Autodesk Fusion 360 part; units mm, degrees
note: some values were not read from the file. Set by a fixed rule: which face or edge a step refers to.
(part 3 of 3)
sketch "Sketch2 (4)" plane through (0, 0, 136) normal (0, 0, 1) x (-1, 0, 0) in component "FrontGlass"
  line L0 (-260.8, 5.2) -> (-260.8, 3)
  line L1 (-260.8, 3) -> (-1.2, 3)
  line L2 (-1.2, 3) -> (-1.2, 5.2)
  line L3 (-1.2, 5.2) -> (-260.8, 5.2)
  line L4 (-260.8, 5.2) -> (-250.8, 5.2) construction
  line L5 (-250.8, 5.2) -> (-248.8, 5.2)
  line L6 (-248.8, 5.2) -> (-248.8, 3)
  line L7 (-248.8, 3) -> (-250.8, 3)
  line L8 (-250.8, 3) -> (-250.8, 5.2)
  line L9 (-1.2, 5.2) -> (-11.2, 5.2) construction
  line L10 (-171.6, 3) -> (-171.6, 5.2)
  line L11 (-171.6, 5.2) -> (-169.6, 5.2)
  line L12 (-169.6, 5.2) -> (-169.6, 3)
  line L13 (-169.6, 3) -> (-171.6, 3)
  line L14 (-92.4, 3) -> (-92.4, 5.2)
  line L15 (-92.4, 5.2) -> (-90.4, 5.2)
  line L16 (-90.4, 5.2) -> (-90.4, 3)
  line L17 (-90.4, 3) -> (-92.4, 3)
  line L18 (-13.2, 3) -> (-13.2, 5.2)
  line L19 (-13.2, 5.2) -> (-11.2, 5.2)
  line L20 (-11.2, 5.2) -> (-11.2, 3)
  line L21 (-11.2, 3) -> (-13.2, 3)
  dimension "d328" = 10
  dimension "d329" = 2
  dimension "d330" = 10
  dimension "d348" = 237.6
  dimension "d349" = 0
  constraint perpendicular L0 L4
  constraint horizontal L5
  constraint vertical L6
  constraint horizontal L7
  constraint vertical L8
  constraint collinear L1 L7
  constraint parallel L3 L9
  constraint coincident L2.end L3.start
  constraint coincident L0.start L3.end
  measures "d328" distance of L0.start L4.end
  measures "d329" distance of L4.end L5.end
  measures "d330" distance of L2.end L9.end
extrude "Extrude2''" add sketch "Sketch2 (4)" along normal blind 1.5 contours L1 L3 L5 L6 L7 L8 | L1 L3 L10 L11 L12 L13 | L1 L3 L14 L15 L16 L17 | L1 L3 L18 L19 L20 L21 bodies 18 in component "FrontGlass"
ref_plane "WorkPlane1" through (131, -4.1, 67.5) normal (0, 0, 1) x (1, 0, 0) in component "FrontGlass"
ref_plane "WorkPlane2" through (131, -4.1, 67.5) normal (1, 0, 0) x (0, 0, -1) in component "FrontGlass"
mirror "Mirror1'" about plane through (131, -4.1, 67.5) normal (0, 0, 1) of "Extrude2''" in component "FrontGlass"
sketch "Sketch3 (4)" plane through (-1, 0, 0) normal (-1, 0, 0) x (0, -1, 0) in component "FrontGlass"
  line L0 (3, 1.2) -> (5.2, 1.2)
  line L1 (5.2, 1.2) -> (5.2, 133.8)
  line L2 (5.2, 133.8) -> (3, 133.8)
  line L3 (3, 133.8) -> (3, 1.2)
  line L4 (5.2, 133.8) -> (5.2, 123.8) construction
  line L5 (5.2, 123.8) -> (3, 123.8)
  line L6 (3, 123.8) -> (3, 121.8)
  line L7 (3, 121.8) -> (5.2, 121.8)
  line L8 (5.2, 121.8) -> (5.2, 123.8)
  line L9 (5.2, 1.2) -> (5.2, 11.2) construction
  line L10 (5.2, 11.2) -> (3, 11.2)
  line L11 (3, 11.2) -> (3, 13.2)
  line L12 (3, 13.2) -> (5.2, 13.2)
  line L13 (5.2, 13.2) -> (5.2, 11.2)
  line L14 (5.2, 121.8) -> (5.2, 13.2) construction
  line L15 (5.2, 68.5) -> (3, 68.5)
  line L16 (3, 68.5) -> (3, 66.5)
  line L17 (3, 66.5) -> (5.2, 66.5)
  line L18 (5.2, 66.5) -> (5.2, 68.5)
  dimension "d335" = 10
  dimension "d336" = 2
  dimension "d337" = 10
  dimension "d338" = 2
  dimension "d341" = 2
  constraint perpendicular L2 L4
  constraint horizontal L5
  constraint vertical L6
  constraint horizontal L7
  constraint vertical L8
  constraint coincident L3 L6.end
  constraint perpendicular L0 L9
  constraint horizontal L10
  constraint vertical L11
  constraint horizontal L12
  constraint vertical L13
  constraint coincident L3 L11.end
  constraint horizontal L15
  constraint vertical L16
  constraint horizontal L17
  constraint vertical L18
  constraint coincident L3 L16.end
  constraint coincident L14 L15.start
  constraint midpoint L3 L16
  constraint coincident L0.end L1.start
  constraint coincident L1.end L2.start
  measures "d335" distance of L1.end L4.end
  measures "d336" distance of L4.end L7.end
  measures "d337" distance of L0.end L9.end
  measures "d338" distance of L9.end L12.end
  measures "d341" distance of L15.start L17.end
extrude "Extrude3'''" add sketch "Sketch3 (4)" along normal blind 1.5 contours L1 L3 L10 L11 L12 L13 | L1 L3 L15 L16 L17 L18 | L1 L3 L5 L6 L7 L8 bodies 18 in component "FrontGlass"
mirror "Mirror2''" about plane through (131, -4.1, 67.5) normal (1, 0, 0) of "Extrude3'''" in component "FrontGlass"
combine "Combine9" operation cut target body 15 tool bodies 18 keep tools in component "Enclosure"
combine "Combine10" operation cut target body 14 tool bodies 18 keep tools in component "Enclosure"
combine "Combine11" operation cut target body 16 tool bodies 18 keep tools in component "Enclosure"
combine "Combine12" operation cut target body 13 tool bodies 18 keep tools in component "Enclosure"
move_face "OffsetFaces6" offset -0.1 56 faces at (249.4667, -3, 137) (249.4667, -4.4667, 137.5) (248.8, -4.4667, 136.5) (250.8, -3.7333, 136.5) (170.2667, -3, 136.5) (171.6, -3.7333, 136.5) (170.2667, -4.4667, 137.5) (169.6, -4.4667, 136.5) (90.4, -4.4667, 136.5) (91.0667, -3, 136.5) (91.7333, -3.7333, 137.5) (92.4, -3.7333, 136.5) (11.2, -4.4667, 136.5) (13.2, -3.7333, 136.5) (11.8667, -3, 137) (12.5333, -3.7333, 137.5) (11.8667, -3, -2) (91.0667, -3, -1.5) (170.2667, -3, -1.5) (249.4667, -3, -1.5) (91.7333, -3.7333, -2.5) (11.8667, -4.4667, -2.5) (170.2667, -4.4667, -2.5) (249.4667, -4.4667, -2.5) (13.2, -3.7333, -1.5) (11.2, -4.4667, -1.5) (92.4, -3.7333, -1.5) (90.4, -4.4667, -1.5) (171.6, -3.7333, -1.5) (169.6, -4.4667, -1.5) (250.8, -3.7333, -1.5) (248.8, -4.4667, -1.5) (-1.5, -4.4667, 123.8) (-2.5, -4.4667, 123.1333) (-1.5, -3, 122.4667) (-1.5, -3.7333, 121.8) (-1.5, -3, 67.1667) (-2.5, -3.7333, 67.1667) (-1.5, -3.7333, 66.5) (-1.5, -4.4667, 68.5) (-1.5, -4.4667, 11.2) (-2.5, -3.7333, 12.5333) (-1.5, -3, 11.8667) (-1.5, -3.7333, 13.2) (263.5, -3, 11.8667) (264.5, -3.7333, 12.5333) (263.5, -4.4667, 11.2) (263.5, -3.7333, 13.2) (263.5, -4.4667, 68.5) (263.5, -3, 67.8333) (264.5, -3.7333, 67.1667) (263.5, -3.7333, 66.5) (263.5, -4.4667, 123.8) (263.5, -3, 123.1333) (264.5, -4.4667, 123.1333) (263.5, -3.7333, 121.8) on bodies 13 14 15 16 in component "Enclosure"
move_face "OffsetFaces7" offset -0.1 84 faces at (230.7, 23.8, 137) (230.7, 22.4, 136.9999) (229.3, 26.6, 136.3333) (230.7, 21.7335, 136.3333) (230.7, 22.4, 136.9999) (227.9, 23.4667, 136.3333) (232.1, 23.4667, 136.3333) (164.7, 22.4, 136.9999) (163.3, 25.2, 137) (163.3, 26.6, 136.3333) (161.9, 23.4667, 136.3333) (166.1, 23.4667, 136.3333) (163.3, 21.7335, 136.3333) (164.7, 22.4, 136.9999) (98.7, 22.4, 136.9999) (97.3, 25.2, 137) (100.1, 23.4667, 136.3333) (98.7, 21.7335, 136.3333) (98.7, 22.4, 136.9999) (95.9, 23.4667, 136.3333) (97.3, 26.6, 136.3333) (29.9, 23.4667, 136.3333) (32.7, 21.7335, 136.3333) (32.7, 22.4, 136.9999) (32.7, 22.4, 136.9999) (32.7, 23.8, 137) (34.1, 23.4667, 136.3333) (31.3, 26.6, 136.3333) (32.7, 26.6, -1.6667) (29.9, 23.4667, -1.3333) (32.7, 21.7335, -1.3333) (31.3, 22.4, -1.9999) (34.1, 23.4667, -1.3333) (32.7, 23.8, -2) (31.3, 22.4, -1.9999) (98.7, 22.4, -1.9999) (97.3, 25.2, -2) (98.7, 21.7335, -1.3333) (98.7, 22.4, -1.9999) (100.1, 23.4667, -1.3333) (98.7, 26.6, -1.6667) (95.9, 23.4667, -1.3333) (164.7, 22.4, -1.9999) (164.7, 25.2, -2) (166.1, 23.4667, -1.3333) (161.9, 23.4667, -1.3333) (163.3, 26.6, -1.3333) (163.3, 21.7335, -1.3333) (164.7, 22.4, -1.9999) (229.3, 22.0667, -1.6665) (229.3, 22.4, -1.9999) (232.1, 23.4667, -1.3333) (230.7, 23.8, -2) (229.3, 22.4, -1.9999) (229.3, 26.6, -1.3333) (227.9, 23.4667, -1.3333) (-1.9999, 22.4, 102.45) (-2, 25.2, 102.45) (-1.3333, 26.6, 101.05) (-1.3333, 21.7335, 101.05) (-1.9999, 22.4, 102.45) (-1.3333, 23.4667, 99.65) (-1.3333, 23.4667, 103.85) (-2, 25.2, 32.55) (-1.9999, 22.4, 33.95) (-1.3333, 26.6, 32.55) (-1.6665, 22.0667, 33.95) (-1.9999, 22.4, 33.95) (-1.3333, 23.4667, 35.35) (-1.3333, 23.4667, 31.15) (264, 25.2, 32.55) (263.9999, 22.4, 32.55) (263.6665, 22.0667, 32.55) (263.9999, 22.4, 32.55) (263.3333, 26.6, 33.95) (263.3333, 23.4667, 31.15) (263.3333, 23.4667, 35.35) (263.9999, 22.4, 102.45) (264, 25.2, 102.45) (263.3333, 23.4667, 103.85) (263.6667, 26.6, 101.05) (263.6665, 22.0667, 102.45) (263.9999, 22.4, 102.45) (263.3333, 23.4667, 99.65) on bodies 13 14 15 16 in component "Enclosure"
component "Display" placed x (1, 0, 0) y (0, 1, 0) z (0, 0, 1) at (0, 0, 0)
component "DisplayMount" placed x (1, 0, 0) y (0, 1, 0) z (0, 0, 1) at (0, 0, 0)
component "PowerSupply" placed x (1, 0, 0) y (0, 1, 0) z (0, 0, 1) at (0, 0, 0)
component "Enclosure" placed x (1, 0, 0) y (0, 1, 0) z (0, 0, 1) at (0, 0, 0)
component "FrontGlass" placed x (1, 0, 0) y (0, 1, 0) z (0, 0, 1) at (0, 0, 0)
equation "DisplayModuleWidth = 65.5 mm"
equation "DisplayModuleHeight = 66.5 mm"
equation "d3 = DisplayModuleWidth"
equation "d4 = DisplayModuleHeight"
equation "d11 = 5 mm + 3.2 mm"
equation "d12 = 5 mm + 3.6 mm"
equation "d27 = DisplayModuleWidth"
equation "d28 = DisplayModuleHeight + 2 mm"
equation "d66 = -DisplayModuleWidth"
equation "DisplayMaskThickness = 0.6 mm"
equation "PlywoodThickness = 3.2 mm"
equation "FrontGlassThickness = 2.2 mm"
equation "d184 = FrontGlassThickness"
equation "d185 = -PlywoodThickness"
equation "d187 = PlywoodThickness"
equation "d190 = 52 mm + PlywoodThickness + FrontGlassThickness"
equation "d192 = PlywoodThickness"
equation "d196 = -( 137 mm + PlywoodThickness * 2 )"
equation "d201 = -PlywoodThickness"
equation "d205 = PlywoodThickness"
equation "d212 = -PlywoodThickness"
equation "d225 = PlywoodThickness / 3"
equation "d282 = FrontGlassThickness"
equation "plywoodTolerance = 0.1 mm"
equation "d284 = -plywoodTolerance"
equation "d285 = -plywoodTolerance"
equation "d286 = -plywoodTolerance"
equation "d350 = -plywoodTolerance"
equation "d357 = -plywoodTolerance"
equation "d358 = PlywoodThickness"
equation "d359 = PlywoodThickness"
equation "d360 = PlywoodThickness"
named bodies: "Body1", "Body1 (1)", "Body1 (2)", "Body1 (3)", "Body1 (4)", "Body1 (5)", "Body1 (6)", "Body1 (7)", "DisplayMountRight", "DisplayMountLeft", "EnclosureLeft", "EnclosurRight", "EnclosureTop", "EnclosureBottom", "EnclosureBack", "DisplayMountConnector"
